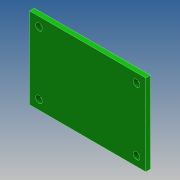
# Autodesk Inventor part: driver motor
Saved by Autodesk Inventor 2017 (Build 210142000, 142)
## iProperties
Part Number: driver motor
Material: Genérico
Document SubType Name: Modeling
Designer: FABLAB
Density: 1 g/cm^3
Appearance: Verde oscuro
Author: FABLAB
Autodesk Inventor part; units mm, degrees
ref_plane "YZ Plane" through (0, 0, 0) normal (1, 0, 0) x (0, 1, 0)
ref_plane "XZ Plane" through (0, 0, 0) normal (0, 1, 0) x (-1, 0, 0)
ref_plane "XY Plane" through (0, 0, 0) normal (0, 0, 1) x (1, 0, 0)
sketch "Boceto1" plane through (0, 0, 0) normal (0, 1, 0) x (-1, 0, 0)
  line L0 (25, 17.5) -> (-25, 17.5)
  line L1 (-25, 17.5) -> (-25, -17.5)
  line L2 (-25, -17.5) -> (25, -17.5)
  line L3 (25, -17.5) -> (25, 17.5)
  line L4 (21, 13.5) -> (-21, 13.5) construction
  line L5 (-21, 13.5) -> (-21, -13.5) construction
  line L6 (-21, -13.5) -> (21, -13.5) construction
  line L7 (21, -13.5) -> (21, 13.5) construction
  circle A0 centre (21, 13.5) radius 1.5
  circle A1 centre (21, -13.5) radius 1.5
  circle A2 centre (-21, -13.5) radius 1.5
  circle A3 centre (-21, 13.5) radius 1.5
  point P0 (0, 0)
  point P1 (25, 0)
  point P2 (0, 17.5)
  dimension "d0" = 3
  dimension "d1" = 4
  dimension "d2" = 35
  dimension "d3" = 50
  constraints: 16 end point, 4 centre point, 4 parallel, 3 coincident, 3 equal radius, 2 midpoint, 2 perpendicular, 1 horizontal, 1 horizontal alignment, 1 vertical alignment, 3 other
  measures "d0" diameter of A0
  measures "d1" distance between parallel lines of L3 L7
  measures "d2" distance of L2.end L0.start
  measures "d3" distance of L0.start L0.end
extrude "Extrusión1" add sketch "Boceto1" along normal blind 2
